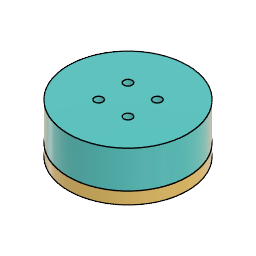
Ear Mount v3 (Autodesk Fusion 360 archive; units mm, degrees)
design "Mitoot 2804"
Autodesk Fusion 360 part; units mm, degrees
sketch "Sketch1" plane through (0, 0, 0) normal (0, 0, 1) x (1, 0, 0)
  circle A0 centre (0, 0) radius 17.25
  line L0 (6.75, -6.75) -> (-6.75, -6.75) construction
  line L1 (-6.75, -6.75) -> (-6.75, 6.75) construction
  line L2 (-6.75, 6.75) -> (6.75, 6.75) construction
  line L3 (6.75, 6.75) -> (6.75, -6.75) construction
  line L4 (6.75, -6.75) -> (-6.75, 6.75) construction
  line L5 (-6.75, -6.75) -> (6.75, 6.75) construction
  dimension "d1" = 34.5
  dimension "d2" = 13.5
  constraint coincident A0.centre origin
  constraint horizontal L0
  constraint perpendicular L0 L1
  constraint parallel L0 L2
  constraint parallel L1 L3
  constraint coincident L4 A0.centre
  constraint coincident L5 A0.centre
  constraint equal L1 L2
  measures "d1" diameter of A0
  measures "d2" distance of L1.end L2.end
extrude "Extrude1" add sketch "Sketch1" along normal blind 3.5 makes body 1
extrude "Extrude2" add 1 faces at (4.4063, 6.4628, 3.5) along direction (0, 0, 1) blind 10.75 separate body on bodies 1 makes body 2
hole "Hole1" at (-6.75, -6.75, 0) at (6.75, -6.75, 0) at (6.75, 6.75, 0) at (-6.75, 6.75, 0) direction (0, 0, 1) diameter 2.9 depth 2 tip angle 180 bodies 1
sketch "Sketch2" plane through (0, 0, 14.25) normal (0, 0, 1) x (-1, 0, 0)
  circle A0 centre (0, 0) radius 17.25
  line L0 (-4.25, 4.25) -> (4.25, 4.25) construction
  line L1 (4.25, 4.25) -> (4.25, -4.25) construction
  line L2 (4.25, -4.25) -> (-4.25, -4.25) construction
  line L3 (-4.25, -4.25) -> (-4.25, 4.25) construction
  line L4 (-4.25, 4.25) -> (4.25, -4.25) construction
  line L5 (4.25, 4.25) -> (-4.25, -4.25) construction
  dimension "d11" = 8.5
  constraint horizontal L0
  constraint perpendicular L0 L1
  constraint parallel L0 L2
  constraint parallel L1 L3
  constraint coincident L4 A0.centre
  constraint coincident L5 A0.centre
  constraint equal L1 L2
  constraint coincident A0.centre origin
  measures "d11" distance of L1.end L2.end
hole "Hole2" at (-4.25, 4.25, 14.25) at (4.25, 4.25, 14.25) at (4.25, -4.25, 14.25) at (-4.25, -4.25, 14.25) direction (0, 0, -1) diameter 2.4 depth 2 tip angle 180 bodies 2
copy_body "Body->Comp1" bodies 1 removing the originals makes body 3 in component "Bottom"
copy_body "Body->Comp2" bodies 2 removing the originals makes body 4 in component "Top"
component "Bottom" placed x (1, 0, 0) y (0, 1, 0) z (0, 0, 1) at (0, 0, 0)
component "Top" placed x (1, 0, 0) y (0, 1, 0) z (0, 0, 1) at (0, 0, 0)
equation "d3 = 3.5 mm"
equation "d8 = 14.25 mm - d3"
